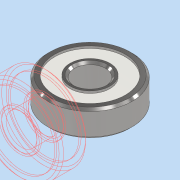
# Autodesk Inventor part: Подшипник
Saved by Autodesk Inventor 2021.2 (Build 252289000, 289)
## iProperties
Created: 2024-11-10
Part Number: Подшипник
Material: Сталь, высокопрочная, низколегированная
Document SubType Name: Modeling
Designer: barko
Density: 5409.93 g/cm^3
Appearance: Сталь — полированная
Mass: 7100 g
Surface Area: 10.1087 cm^2
Volume: 1.3124 cm^3
Author: barko
Autodesk Inventor part; units mm, degrees
ref_plane "YZ Plane" through (0, 0, 0) normal (1, 0, 0) x (0, 1, 0)
ref_plane "XZ Plane" through (0, 0, 0) normal (0, 1, 0) x (-1, 0, 0)
ref_plane "XY Plane" through (0, 0, 0) normal (0, 0, 1) x (1, 0, 0)
sketch "Эскиз1" plane through (0, 0, 0) normal (0, 1, 0) x (-1, 0, 0)
  circle A0 centre (0, 0) radius 9.5
  circle A1 centre (0, 0) radius 3.5
  circle A2 centre (0, 0) radius 8
  circle A3 centre (0, 0) radius 4.5
  dimension "d0" = 19
  dimension "d3" = 7
  dimension "d4" = 1.5
  dimension "d5" = 1
  constraints: 4 centre point, 4 coincident
  measures "d0" diameter of A0
  measures "d3" diameter of A1
  measures "d4" radial gap between concentric circles of A2 A0
  measures "d5" radial gap between concentric circles of A1 A3
extrude "Выдавливание1" add sketch "Эскиз1" along normal mid plane 6
extrude "Выдавливание2" add sketch "Эскиз1" along normal mid plane 5 contours A2
chamfer "Фаска1" distance 0.5 angle 45 4 edges at (9.5, -3, 0) (9.5, 3, 0) (3.5, -3, 0) (3.5, 3, 0)
equation "\"d0\" = bearing_outer"
equation "\"d3\" = bearing_inner"
equation "\"d6\" = bearing_width"
equation "\"blade_radius\" = 127"
equation "\"bearing_inner\" = 7"
equation "\"bearing_outer\" = 19"
equation "\"bearing_width\" = 6"
equation "\"beam_length\" = 254"
equation "\"motor_height\" = 24"
equation "\"motor_diameter\" = 28"
equation "\"motor_blade_offset\" = 2"
equation "\"M4_nut_lock_width\" = 6.8"
equation "\"M4_screw_innerHex_cap_diam\" = 6.6"
equation "\"M4_screw_innerHex_cap_height\" = 4"
equation "\"M4_nut_lock_height\" = 5"
